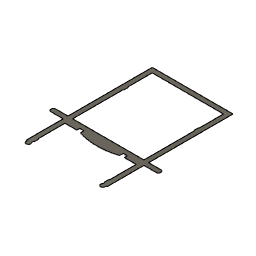
3F廊下用平面[少し幅大きく作ったから修正入れていこう] (Autodesk Fusion 360 design; units mm, degrees)
Autodesk Fusion 360 part; units mm, degrees
sketch "スケッチ1" plane through (0, 0, 0) normal (0, 0, 1) x (1, 0, 0)
  line L0 (10000, 0) -> (11000, 0)
  line L1 (11000, -4000) -> (0, -4000)
  line L2 (-63500, -29000.036) -> (-64000, -29000.036)
  line L3 (-63500, 42500) -> (-63500, 46500)
  line L4 (-54000, -6500.036) -> (-54000, -4000)
  line L5 (-64000, -34500.036) -> (-64000, -33000.036)
  line L6 (-34000, 2000) -> (-34000, -2000)
  arc A0 (-79000, 0) -> (-79000, -4000) centre (-78000, -2000) ccw
  line L7 (-67000, -35000) -> (-68000, -35000)
  line L8 (-64000, -6500.036) -> (-64000, -29000.036)
  line L9 (-64000, 0) -> (-34000, 0)
  line L10 (-64000, 42500) -> (-63500, 42500)
  line L11 (0, 41000) -> (0, 43977.4822)
  line L12 (-4500, -33000.036) -> (-4500, -29000.036)
  arc A1 (-67000, -35000) -> (-64000, -34500.036) centre (-65310.0198, -35889.9814) ccw
  arc A2 (11000, -4000) -> (11000, 0) centre (10000, -2000) ccw
  line L13 (-79000, -4000) -> (-68000, -4000)
  line L14 (-68000, 41000) -> (-68000, 43977.4822)
  line L15 (11000, -4000) -> (0, -4000)
  line L16 (-1000, -35000) -> (0, -35000)
  line L17 (-64000, 0) -> (-64000, 42500)
  line L18 (-78000, 0) -> (-79000, 0)
  line L19 (-68000, 0) -> (-78000, 0)
  line L20 (-4000, 0) -> (-4000, 42500)
  line L21 (-64000, -6500.036) -> (-54000, -6500.036)
  line L22 (-14000, -6500.036) -> (-14000, -4000)
  line L23 (-68000, 0) -> (-68000, 41000)
  line L24 (-63500, -33000.036) -> (-63500, -29000.036)
  line L25 (-4000, 0) -> (-34000, 0)
  line L26 (-4000, -6500.036) -> (-14000, -6500.036)
  line L27 (-4000, -33000.036) -> (-4500, -33000.036)
  line L28 (-4000, 42500) -> (-4500, 42500)
  line L29 (-68000, -4000) -> (-68000, -35000)
  line L30 (11000, 0) -> (0, 0)
  line L31 (-64000, -33000.036) -> (-63500, -33000.036)
  line L32 (0, -4000) -> (0, -35000)
  line L33 (-4500, 46500) -> (-4000, 46500)
  line L34 (0, 0) -> (10000, 0)
  line L35 (-63500, 46500) -> (-64000, 46500)
  line L36 (-4000, -34500.036) -> (-4000, -33000.036)
  line L37 (-4000, -6500.036) -> (-4000, -29000.036)
  line L38 (-4500, -29000.036) -> (-4000, -29000.036)
  line L39 (-4500, 42500) -> (-4500, 46500)
  arc A3 (-4000, -34500.036) -> (-1000, -35000) centre (-2689.9802, -35889.9814) ccw
  line L40 (0, 0) -> (0, 41000)
  line L41 (-54000, -4000) -> (-50500, -4000)
  line L42 (-50500, -4000) -> (-50500, -7000)
  line L43 (-14000, -4000) -> (-17500, -4000)
  line L44 (-17500, -4000) -> (-17500, -7000)
  arc A4 (-50500, -7000) -> (-17500, -7000) centre (-34000, 44124.3719) ccw
  line L45 (-68000, 71000) -> (-68000, 43977.4822)
  line L46 (-64000, 67000) -> (-4000, 67000)
  line L47 (0, 71000) -> (-68000, 71000)
  line L48 (0, 43977.4822) -> (0, 71000)
  line L49 (-4000, 67000) -> (-4000, 47000)
  line L50 (-4000, 46500) -> (-4000, 47000)
  line L51 (-64000, 67000) -> (-64000, 46500)
  point P0 (-64000, 42500)
  point P1 (-64000, -6500.036)
  point P2 (-64000, 0)
  point P3 (-64000, -34500.036)
  point P4 (-68000, 0)
  point P5 (-64000, -35000)
  point P6 (-4000, 0)
  point P7 (-64000, 41000)
  point P8 (-4000, -35000)
  point P9 (-4000, 41000)
  point P10 (-4000, -6500.036)
  point P11 (-64000, 0)
  point P12 (-4000, 42500)
  point P13 (-4000, -34500.036)
  constraint perpendicular L4 L41
  constraint perpendicular L41 L42
  constraint perpendicular L22 L43
  constraint perpendicular L43 L44
  constraint perpendicular L45 L47
  constraint perpendicular L46 L51
extrude "押し出し1" add sketch "スケッチ1" along normal blind 10
